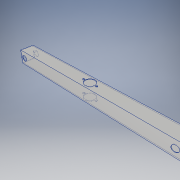
# Autodesk Inventor part: Crossbeam
Saved by Autodesk Inventor 2019 (Build 230136000, 136)
## iProperties
Created: 2018-09-28
Part Number: Crossbeam
Material: Aluminum 6061
Document SubType Name: Modeling
Designer: Adhik
Density: 2.7 g/cm^3
Appearance: Aluminum - Flat
Mass: 279.491 g
Surface Area: 1314.15 cm^2
Volume: 103.515 cm^3
Author: Adhik
Autodesk Inventor part; units mm, degrees
ref_plane "YZ Plane" through (0, 0, 0) normal (1, 0, 0) x (0, 1, 0)
ref_plane "XZ Plane" through (0, 0, 0) normal (0, 1, 0) x (-1, 0, 0)
ref_plane "XY Plane" through (0, 0, 0) normal (0, 0, 1) x (1, 0, 0)
sketch "Sketch2" plane through (0, 0, 0) normal (1, 0, 0) x (0, 1, 0)
  line L0 (0, -26.67) -> (0, 26.67) construction
  line L1 (-26.67, 0) -> (26.67, 0) construction
  line L2 (17.4625, 17.4625) -> (-17.4625, 17.4625)
  line L3 (-17.4625, 17.4625) -> (-17.4625, -17.4625)
  line L4 (-17.4625, -17.4625) -> (17.4625, -17.4625)
  line L5 (17.4625, -17.4625) -> (17.4625, 17.4625)
  line L6 (19.05, 19.05) -> (-19.05, 19.05)
  line L7 (-19.05, 19.05) -> (-19.05, -19.05)
  line L8 (-19.05, -19.05) -> (19.05, -19.05)
  line L9 (19.05, -19.05) -> (19.05, 19.05)
  point P0 (0, 0)
  point P1 (0, 19.05)
  point P2 (0, 17.4625)
  point P3 (17.4625, 0)
  point P4 (19.05, 0)
  dimension "d0" = 1.5875
  dimension "d1" = 38.1
  constraints: 16 end point, 4 midpoint, 4 parallel, 4 perpendicular, 4 point on line, 2 horizontal
  measures "d0" distance between parallel lines of L6 L2
  measures "d1" distance of L6.start L6.end
extrude "Extrusion1" add sketch "Sketch2" along normal mid plane 457.2
sketch "Sketch3" plane through (-228.6, -19.05, 19.05) normal (0, 0, 1) x (1, 0, 0)
  line L0 (-91.44, 19.05) -> (548.64, 19.05) construction
  line L1 (228.6, -7.62) -> (228.6, 45.72) construction
  circle A0 centre (12.7, 19.05) radius 7.9375
  line L2 (0, 0) -> (0, 38.1) construction
  circle A1 centre (444.5, 19.05) radius 7.9375
  point P0 (228.6, 19.05)
  dimension "d4" = 12.7
  dimension "d5" = 15.875
  constraints: 2 centre point, 1 point on line, 1 symmetric about line, 1 other
  measures "d4" distance from line of L2 A0.centre
  measures "d5" diameter of A0
extrude "Extrusion2" cut sketch "Sketch3" against normal through all
sketch "Sketch5" plane through (-228.6, 19.05, 19.05) normal (0, 1, 0) x (1, 0, 0)
  circle A0 centre (228.6, 19.05) radius 14.2875
  dimension "d11" = 28.575
  constraints: 1 centre point, 1 coincident
  measures "d11" diameter of A0
extrude "Extrusion4" cut sketch "Sketch5" against normal through all
sketch "Sketch6" plane through (-228.6, 19.05, 19.05) normal (0, 1, 0) x (1, 0, 0)
  line L0 (-91.44, 19.05) -> (548.64, 19.05) construction
  line L1 (228.6, 45.72) -> (228.6, -7.62) construction
  circle A0 centre (209.55, 19.05) radius 3.175 construction
  circle A1 centre (247.65, 19.05) radius 3.175 construction
  circle A2 centre (228.6, 19.05) radius 15.875 construction
  circle A3 centre (209.55, 19.05) radius 2.667
  circle A4 centre (247.65, 19.05) radius 2.667
  dimension "d14" = 31.75
  dimension "d15" = 6.35
  dimension "d16" = 5.334
  constraints: 5 centre point, 3 coincident, 2 point on line, 1 equal radius, 1 tangent, 1 other
  measures "d14" diameter of A2
  measures "d15" diameter of A0
  measures "d16" diameter of A3
extrude "Extrusion5" cut sketch "Sketch6" against normal through all
body "Solid1"
